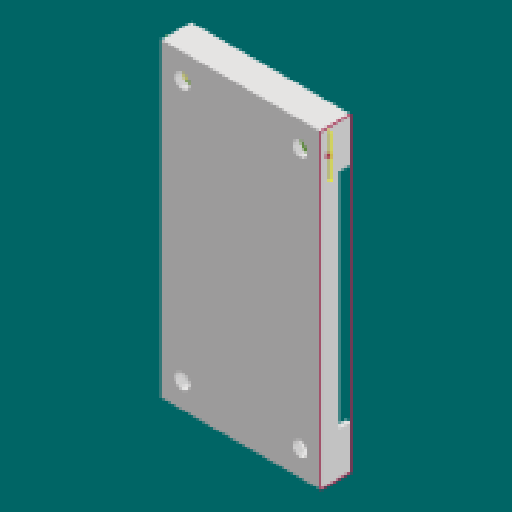
# Autodesk Inventor part: bawah
Saved by Autodesk Inventor 2025.2 (Build 292293000, 293)
## iProperties
Created: 2025-04-22
Part Number: bawah
Material: Generic
Document SubType Name: Modeling
Designer: ia088
Density: 1 g/cm^3
Appearance: Default
Author: ia088
Autodesk Inventor part; units mm, degrees
ref_plane "YZ Plane" through (0, 0, 0) normal (1, 0, 0) x (0, 1, 0)
ref_plane "XZ Plane" through (0, 0, 0) normal (0, 1, 0) x (-1, 0, 0)
ref_plane "XY Plane" through (0, 0, 0) normal (0, 0, 1) x (1, 0, 0)
ref_plane "Work Plane1" through (0, 0, 0) normal (0, 0, 1) x (1, 0, 0)
sketch "Sketch1" plane through (0, 0, 0) normal (0, 0, 1) x (1, 0, 0)
  circle A0 centre (39.1667, -0.7223) radius 5 projected
  circle A1 centre (-39.1667, -0.7223) radius 5 projected
  line L0 (-50, -13) -> (-28.3333, -13) projected
  line L1 (-28.3333, -13) -> (-28.3333, 10) projected
  line L2 (-28.3333, 10) -> (28.3333, 10) projected
  line L3 (28.3333, -13) -> (28.3333, 10) projected
  line L4 (28.3333, -13) -> (50, -13) projected
  line L5 (50, -13) -> (50, 13) projected
  line L6 (50, 13) -> (-50, 13) projected
  line L7 (-50, 13) -> (-50, -13) projected
  line L8 (28.3333, -161) -> (31.3333, -161) projected
  line L9 (31.3333, -161) -> (31.3333, -13) projected
  line L10 (31.3333, -13) -> (28.3333, -13) projected
  line L11 (28.3333, -13) -> (28.3333, -161) projected
  circle A2 centre (39.1667, -173.2777) radius 5 projected
  circle A3 centre (-39.1667, -173.2777) radius 5 projected
  line L12 (50, -161) -> (28.3333, -161) projected
  line L13 (28.3333, -161) -> (28.3333, -184) projected
  line L14 (28.3333, -184) -> (-28.3333, -184) projected
  line L15 (-28.3333, -161) -> (-28.3333, -184) projected
  line L16 (-28.3333, -161) -> (-50, -161) projected
  line L17 (-50, -161) -> (-50, -187) projected
  line L18 (-50, -187) -> (50, -187) projected
  line L19 (50, -187) -> (50, -161) projected
  line L20 (-31.3333, -161) -> (-28.3333, -161) projected
  line L21 (-28.3333, -161) -> (-28.3333, -13) projected
  line L22 (-28.3333, -13) -> (-31.3333, -13) projected
  line L23 (-31.3333, -13) -> (-31.3333, -161) projected
  line L24 (-31.3333, -161) -> (-28.3333, -161) projected
  line L25 (-28.3333, -161) -> (-28.3333, -13) projected
  line L26 (-28.3333, -13) -> (-31.3333, -13) projected
  line L27 (-31.3333, -13) -> (-31.3333, -161) projected
  line L28 (53, 16) -> (-53, 16)
  line L29 (-53, 16) -> (-53, -187)
  line L30 (53, -187) -> (53, 16)
  line L31 (53, 16) -> (-53, -187) construction
  line L32 (-53, 16) -> (53, -187) construction
  line L33 (53, -187) -> (53, -190)
  line L34 (53, -190) -> (-53, -190)
  line L35 (-53, -190) -> (-53, -187)
  point P0 (0, 0)
  point P1 (0, -85.5)
  dimension "d0" = 106
  dimension "d1" = 203
  dimension "d2" = 3
  constraints: 16 end point, 3 perpendicular, 2 midpoint, 1 horizontal, 1 parallel, 1 vertical
  measures "d0" distance of L30.start L29.end
  measures "d1" distance of L30.start L28.start
  measures "d2" distance of L30.start L33.end
extrude "Extrusion1" add sketch "Sketch1" along normal blind 5 contours L7 L6 L5 L4 L3 L2 L1 L0 | L0 L21 L16 L23 | L1 L2 L3 L11 L13 L14 L15 L21 | L16 L15 L14 L13 L8 L12 L19 L18 L17 | L9 L8 L11 L4 | L30 L33 L34 L35 L29 L28
sketch "Sketch2" plane through (0, 0, 0) normal (0, 0, -1) x (-1, 0, 0)
  line L0 (-53, 16) -> (53, 16) projected
  line L1 (-53, -190) -> (-53, 16) projected
  line L2 (53, -190) -> (-53, -190) projected
  line L3 (53, 16) -> (53, -190) projected
  line L4 (-50, 13) -> (50, 13)
  line L5 (50, 13) -> (50, -187)
  line L6 (50, -187) -> (-50, -187)
  line L7 (-50, -187) -> (-50, 13)
  point P0 (0, 0)
  dimension "d5" = 3
  constraints: 8 end point, 3 other
  measures "d5" distance between parallel lines of L1 L7
extrude "Extrusion2" add sketch "Sketch2" along normal blind 15
sketch "Sketch3" plane through (53, -190, 5) normal (1, 0, 0) x (0, 0, -1)
  line L0 (0, 206) -> (20, 206) projected
  line L1 (0, 0) -> (0, 206) projected
  line L2 (20, 0) -> (0, 0) projected
  line L3 (20, 206) -> (20, 0) projected
  point P0 (5, 190)
sketch "Sketch4" plane through (53, -190, 5) normal (1, 0, 0) x (0, 0, -1)
  line L0 (0, 0) -> (0, 206) projected
  line L1 (20, 206) -> (20, 0) projected
  line L2 (5, 177) -> (58, 177) projected
  line L3 (20, 177) -> (0, 177)
  line L4 (58, 29) -> (5, 29) projected
  line L5 (20, 29) -> (0, 29)
  line L6 (12.6827, 177) -> (12.6827, 29)
  point P0 (5, 190)
  constraints: 10 point on line, 6 end point, 1 perpendicular
extrude "Extrusion3" cut sketch "Sketch4" against normal up to surface (106 mm away) contours L6 L2 L1 L4
body "Solid1"
